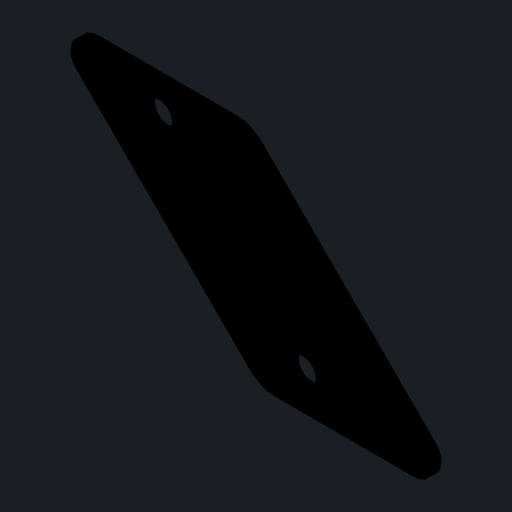
# Autodesk Inventor part: chrissled
Saved by Autodesk Inventor 2024.2 (Build 282272000, 272)
## iProperties
Created: 2024-01-18
Part Number: chrissled
Material: Polycarbonate, Clear
Document SubType Name: Sheet Metal
Designer: reima
Density: 1.2 g/cm^3
Appearance: Anodized - Black
Flat Pattern Width: 0.15875 cm
Flat Pattern Length: 6.40447 cm
Flat Pattern Area: 1.01671 cm^2
Sheet Metal Rule: Default
Sheet Metal Width: 0.063 in
Sheet Metal Length: 2.521 in
Sheet Metal Area: 0.158 in^2
Author: reima
Autodesk Inventor part; units mm, degrees
ref_plane "YZ Plane" through (0, 0, 0) normal (1, 0, 0) x (0, 1, 0)
ref_plane "XZ Plane" through (0, 0, 0) normal (0, 1, 0) x (-1, 0, 0)
ref_plane "XY Plane" through (0, 0, 0) normal (0, 0, 1) x (1, 0, 0)
sketch "Sketch2" plane through (0, 0, 0) normal (0, 0, 1) x (1, 0, 0)
  circle A0 centre (-57.15, -7.5944) radius 2.3114 projected
  circle A1 centre (-44.45, -7.5944) radius 2.3114 projected
  circle A2 centre (-31.75, -34.1628) radius 2.3114 projected
  circle A3 centre (0.0154, -27.8287) radius 41.275 construction
  line L0 (-52.827, -2.4128) -> (-63.5, -2.4128) projected
  line L1 (-41.0824, -38.6529) -> (-71.9025, -7.8329)
  circle A4 centre (-63.5, -15.1128) radius 0.7938 construction
  circle A5 centre (-38.1, -40.5128) radius 0.7937 construction
  line L2 (-36.5923, -40.5128) -> (-11.9627, -40.5128)
  line L3 (-69.6574, -2.4128) -> (-45.0278, -2.4128)
  line L4 (-40.5377, -4.2727) -> (-9.7176, -35.0927)
  arc A6 (-69.6574, -2.4128) -> (-71.9025, -7.8329) centre (-69.6574, -5.5878) ccw
  arc A7 (-11.9627, -40.5128) -> (-9.7176, -35.0927) centre (-11.9627, -37.3378) ccw
  arc A8 (-40.5377, -4.2727) -> (-45.0278, -2.4128) centre (-45.0278, -8.7628) ccw
  arc A9 (-41.0824, -38.6529) -> (-36.5923, -40.5128) centre (-36.5923, -34.1628) ccw
  point P0 (-39.2225, -40.5128)
  point P1 (-77.3225, -2.4128)
  point P2 (-4.2975, -40.5128)
  point P3 (-42.3975, -2.4128)
  dimension "d19" = 1.5875
  dimension "d20" = 1.5875
  dimension "d21" = 34.925
  dimension "d22" = 34.925
  dimension "d23" = 3.175
  dimension "d24" = 6.35
  dimension "d25" = 6.35
  dimension "d28" = 82.55
  dimension "d29" = 38.1
  dimension "d30" = 25.4159
  dimension "d31" = 0
  dimension "d32" = 0
  dimension "d33" = 12.0187
  dimension "d34" = 7.3747
  dimension "d35" = 14.9217
  constraints: 11 tangent, 8 end point, 8 point on circle, 8 point on line, 7 centre point, 2 coincident, 2 horizontal, 1 equal radius, 3 other
  measures "d19" diameter of A4
  measures "d20" diameter of A5
  measures "d21" distance of point (-39.223, -40.513) point (-4.298, -40.513)
  measures "d22" distance of point (-77.323, -2.413) point (-42.398, -2.413)
  measures "d23" radius of A6
  measures "d24" radius of A8
  measures "d25" radius of A9
  measures "d28" diameter of A3
  measures "d29" distance between parallel lines of L2 L0
  measures "d30" distance from line of A3.centre L0
  measures "d31" distance from line of point (-52.827, -2.413) L0
  measures "d32" distance from line of point (-63.5, -2.413) L0
  measures "d33" distance from line of A3.centre L4
  measures "d34" distance from line of point (-52.827, -2.413) L4
  measures "d35" distance from line of point (-63.5, -2.413) L4
extrude "Extrusion2" add sketch "Sketch2" along normal blind 1.5875 contours A1 | L3 A8 L4 A7 L2 A9 L1 A6 L0
sketch "Sketch3" plane through (0, 0, 1.5875) normal (0, 0, 1) x (1, 0, 0)
  line L0 (-71.9025, -7.8329) -> (-41.0824, -38.6529)
  arc A0 (-41.0824, -38.6529) -> (-36.5923, -40.5128) centre (-36.5923, -34.1628) ccw
  line L1 (-36.5923, -40.5128) -> (-11.9627, -40.5128)
  arc A1 (-11.9627, -40.5128) -> (-9.7176, -35.0927) centre (-11.9627, -37.3378) ccw
  line L2 (-9.7176, -35.0927) -> (-40.5377, -4.2727)
  arc A2 (-40.5377, -4.2727) -> (-45.0278, -2.4128) centre (-45.0278, -8.7628) ccw
  line L3 (-45.0278, -2.4128) -> (-69.6574, -2.4128)
  arc A3 (-69.6574, -2.4128) -> (-71.9025, -7.8329) centre (-69.6574, -5.5878) ccw
  circle A4 centre (-31.75, -34.1628) radius 2.3114
  circle A5 centre (-57.15, -7.5944) radius 2.3114
  point P0 (0, 0)
sheet face with bend "Face1" sketch "Sketch3" thickness 1.5875 toward (0, 0, -1) bend radius 1.5875 relief straight relief width 1.5875 relief depth 0.7937
bend "Bend1"
equation "\"d36\" = Thickness"
equation "\"d37\" = BendRadius"
equation "\"d38\" = BendReliefWidth"
equation "\"d40\" = MinimumRemnant"
equation "\"d39\" = BendReliefDepth"
equation "\"d41\" = TransitionRadius"
equation "\"BendRadius\" = Thickness"
equation "\"BendReliefWidth\" = Thickness"
equation "\"BendReliefDepth\" = 0.5 * Thickness"
equation "\"CornerReliefSize\" = 4 * Thickness"
equation "\"MinimumRemnant\" = 2 * Thickness"
equation "\"TransitionRadius\" = BendRadius"
equation "\"JacobiRadiusSize\" = BendRadius"
equation "\"GapSize\" = Thickness"
equation "\"Thickness\" = 1.5875"
body "Solid2"
